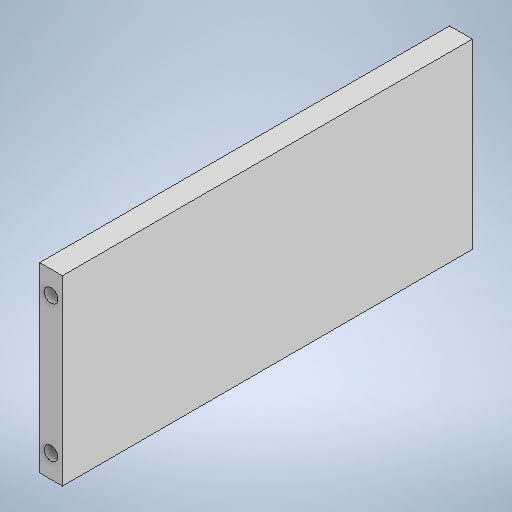
# Autodesk Inventor part: Frontal
Saved by Autodesk Inventor 2025.2 (Build 292293000, 293)
## iProperties
Created: 2025-01-27
Part Number: Frontal
Material: Genérico
Document SubType Name: Modeling
Designer: alex
Density: 1 g/cm^3
Appearance: Valor por defecto
Author: alex
Autodesk Inventor part; units mm, degrees
ref_plane "YZ Plane" through (0, 0, 0) normal (1, 0, 0) x (0, 1, 0)
ref_plane "XZ Plane" through (0, 0, 0) normal (0, 1, 0) x (-1, 0, 0)
ref_plane "XY Plane" through (0, 0, 0) normal (0, 0, 1) x (1, 0, 0)
sketch "Boceto1" plane through (0, 0, 0) normal (1, 0, 0) x (0, 1, 0)
  line L0 (0, 0) -> (40, 0)
  line L1 (40, 0) -> (40, -90)
  line L2 (40, -90) -> (0, -90)
  line L3 (0, -90) -> (0, 0)
  dimension "d0" = 40
  dimension "d1" = 90
  constraints: 8 end point, 2 parallel, 1 horizontal, 1 perpendicular
  measures "d0" distance of L1.end L2.end
  measures "d1" distance of L0.end L1.end
extrude "Extrusión1" add sketch "Boceto1" along normal blind 5
sketch "Boceto2" plane through (0, 0, 0) normal (0, 0, 1) x (1, 0, 0)
  circle A0 centre (2.5, 5) radius 1.5
  circle A1 centre (2.5, 35) radius 1.5
  line L0 (0, 40) -> (0, 0) projected
  line L1 (0, 40) -> (5, 40) projected
  line L2 (0, 0) -> (5, 0) projected
  line L3 (5, 40) -> (5, 0) projected
  point P0 (2.5, 0)
  dimension "d4" = 3
  dimension "d5" = 3
  dimension "d6" = 2.5
  dimension "d7" = 5
  dimension "d8" = 5
  dimension "d9" = 2.5
  constraints: 2 centre point, 1 midpoint
  measures "d4" diameter of A0
  measures "d5" diameter of A1
  measures "d6" distance from line of L0 A1.centre
  measures "d7" distance from line of L1 A1.centre
  measures "d8" distance of point (2.5, 0) A0.centre
  measures "d9" distance from line of L3 A0.centre
extrude "Extrusión2" cut sketch "Boceto2" against normal blind 3 contours A0 | A1
sketch "Boceto3" plane through (0, 0, -90) normal (0, 0, -1) x (-1, 0, 0)
  circle A0 centre (-2.5, 5) radius 1.5 projected
  circle A1 centre (-2.5, 5) radius 1.5
  circle A2 centre (-2.5, 35) radius 1.5 projected
  circle A3 centre (-2.5, 35) radius 1.5
  point P0 (0, 0)
  constraints: 2 centre point, 2 coincident
extrude "Extrusión3" cut sketch "Boceto3" against normal blind 3
